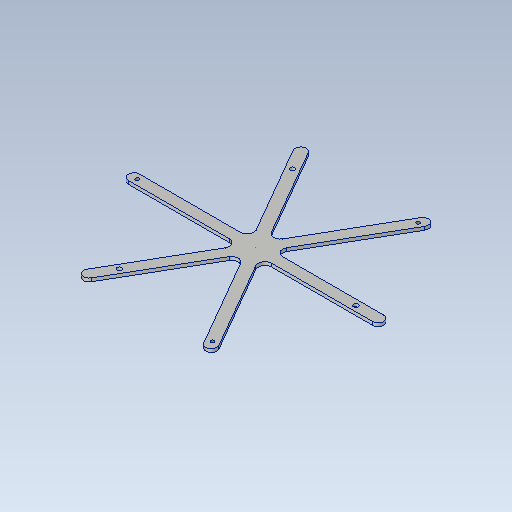
# Autodesk Inventor part: SpiderPrimaryMirror
Saved by Autodesk Inventor 2020 (Build 240168000, 168)
## iProperties
Created: 2019-04-25
Part Number: SpiderPrimaryMirror
Material: Aluminium 6061
Document SubType Name: Modeling
Designer: barto
Density: 2.7 g/cm^3
Appearance: Aluminium — płaski
Author: barto
Autodesk Inventor part; units mm, degrees
ref_plane "YZ Plane" through (0, 0, 0) normal (1, 0, 0) x (0, 1, 0)
ref_plane "XZ Plane" through (0, 0, 0) normal (0, 1, 0) x (-1, 0, 0)
ref_plane "XY Plane" through (0, 0, 0) normal (0, 0, 1) x (1, 0, 0)
sketch "Szkic1" plane through (0, 0, 0) normal (0, 1, 0) x (-1, 0, 0)
  line L0 (-115, -5) -> (115, -5)
  line L1 (115, -5) -> (115, 5)
  line L2 (115, 5) -> (-115, 5)
  line L3 (-115, 5) -> (-115, -5)
  line L4 (-53.1699, -102.0929) -> (61.8301, 97.0929)
  line L5 (53.1699, 102.0929) -> (-61.8301, -97.0929)
  line L6 (-61.8301, -97.0929) -> (-53.1699, -102.0929)
  line L7 (61.8301, 97.0929) -> (53.1699, 102.0929)
  line L8 (61.8301, -97.0929) -> (-53.1699, 102.0929)
  line L9 (-61.8301, 97.0929) -> (53.1699, -102.0929)
  line L10 (53.1699, -102.0929) -> (61.8301, -97.0929)
  line L11 (-53.1699, 102.0929) -> (-61.8301, 97.0929)
  line L12 (115, 5) -> (-115, 5)
  line L13 (-115, -5) -> (115, -5)
  line L14 (115, -5) -> (115, 5)
  line L15 (-115, 5) -> (-115, -5)
  line L16 (53.1699, 102.0929) -> (-61.8301, -97.0929)
  line L17 (-53.1699, -102.0929) -> (61.8301, 97.0929)
  line L18 (61.8301, 97.0929) -> (53.1699, 102.0929)
  line L19 (-61.8301, -97.0929) -> (-53.1699, -102.0929)
  line L20 (-61.8301, 97.0929) -> (53.1699, -102.0929)
  line L21 (61.8301, -97.0929) -> (-53.1699, 102.0929)
  line L22 (-53.1699, 102.0929) -> (-61.8301, 97.0929)
  line L23 (53.1699, -102.0929) -> (61.8301, -97.0929)
  point P0 (0, 0)
  dimension "d6" = 10
  dimension "d7" = 5
  dimension "d8" = 230
  dimension "d9" = 115
  dimension "d12" = 360
  constraints: 48 end point, 49 other
  measures "d6" distance between parallel lines of L2 L0
  measures "d7" distance from line of L2 point (0, 0)
  measures "d8" distance of L0.start L0.end
  measures "d9" distance from line of point (0, 0) L3
extrude "Wyciągnięcie proste2" add sketch "Szkic1" along normal blind 3
sketch "Szkic2" plane through (0, 0, 0) normal (0, -1, 0) x (1, 0, 0)
  line L0 (-53.1699, 102.0929) -> (0, 10) projected
  line L1 (-61.8301, 97.0929) -> (-53.1699, 102.0929) projected
  point P0 (0, 0)
  point P1 (-45, 77.9423)
  point P2 (-45, -77.9423)
  point P3 (90, 0)
  dimension "d48" = 360
  constraints: 4 other
fillet "Zaokrąglenie3" radius 6 6 edges at (8.6603, 1.5, 5) (0, 1.5, 10) (-8.6603, 1.5, 5) (-8.6603, 1.5, -5) (0, 1.5, -10) (8.6603, 1.5, -5)
fillet "Zaokrąglenie4" radius 5 2 edges at (-53.1699, 1.5, 102.0929) (-61.8301, 1.5, 97.0929)
sketch "Szkic3" plane through (0, 0, 0) normal (0, -1, 0) x (1, 0, 0)
  point P0 (0, 0)
  point P1 (0, 0)
  constraints: 1 coincident
pattern_circular "Szyk kołowy1" count 6 over 360 about axis through (0, 0, 0) along (0, -1, 0) of "Zaokrąglenie4"
hole "Otwór1" at (-45, 0, 77.9423) at (-45, 0, -77.9423) at (90, 0, 0) direction (0, 1, 0) diameter 4.5 end through all clearance for "Śruba ze łbem stożkowym ISO 2009/7046" size "M4" standard "ISO"
sketch "Szkic4" plane through (0, 0, 0) normal (0, -1, 0) x (1, 0, 0)
  circle A0 centre (0, 0) radius 106.9
  line L0 (0, 0) -> (-125.8998, 0)
  point P0 (-106.9, 0)
  point P1 (53.45, -92.5781)
  point P2 (53.45, 92.5781)
  dimension "d57" = 213.8
  dimension "d60" = 360
  constraints: 2 end point, 1 coincident, 1 horizontal, 1 horizontal alignment, 1 point on line, 6 other
hole "Otwór2" at (-106.9, 0, 0) at (53.45, 0, -92.5781) at (53.45, 0, 92.5781) direction (0, 1, 0) diameter 3.242 end through all thread size "M4x0.7" class "6H" standard "ISO Metric profile"
chamfer "Faza1" distance 0.4 angle 45 6 edges at (53.45, 0, -90.9571) (90, 0, 2.25) (-45, 0, -75.6923) (-106.9, 0, 1.621) (-45, 0, 80.1923) (53.45, 0, 94.1991)
